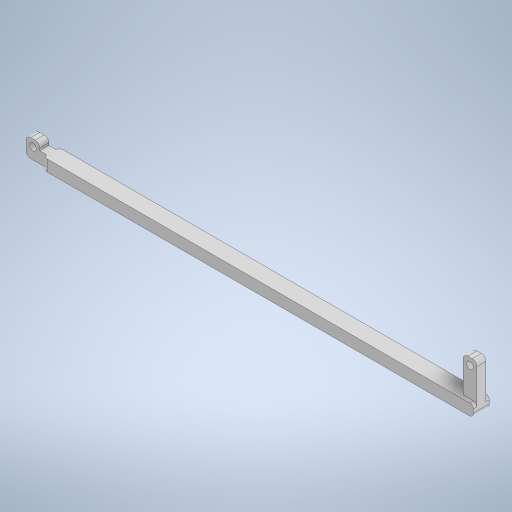
# Autodesk Inventor part: Brace_unequal
Saved by Autodesk Inventor 2024.3 (Build 283343000, 343)
## iProperties
Created: 2024-11-11
Part Number: Brace_unequal
Material: Generic
Document SubType Name: Modeling
Designer: magn1
Density: 1 g/cm^3
Appearance: Default
Author: magn1
Autodesk Inventor part; units mm, degrees
ref_plane "YZ Plane" through (0, 0, 0) normal (1, 0, 0) x (0, 1, 0)
ref_plane "XZ Plane" through (0, 0, 0) normal (0, 1, 0) x (-1, 0, 0)
ref_plane "XY Plane" through (0, 0, 0) normal (0, 0, 1) x (1, 0, 0)
sketch "Sketch1" plane through (0, 0, 0) normal (0, 1, 0) x (-1, 0, 0)
  line L0 (99.05, 3.5) -> (-99.05, 3.5)
  line L1 (-99.05, 3.5) -> (-99.05, -3.5)
  line L2 (-99.05, -3.5) -> (99.05, -3.5)
  line L3 (99.05, -3.5) -> (99.05, 3.5)
  line L4 (99.05, 3.5) -> (-99.05, -3.5) construction
  line L5 (-99.05, 3.5) -> (99.05, -3.5) construction
  point P0 (0, 0)
  dimension "d0" = 198.1
  dimension "d1" = 7
  constraints: 12 end point, 2 midpoint, 2 parallel, 1 horizontal, 1 perpendicular
  measures "d0" distance of L2.end L1.end
  measures "d1" distance of L1.end L0.end
extrude "Extrusion1" add sketch "Sketch1" along normal blind 5
sketch "Sketch2" plane through (0, 5, 0) normal (0, 1, 0) x (1, 0, 0)
  line L0 (99.05, -3.5) -> (99.05, 3.5) projected
  line L1 (99.05, 2) -> (93.05, 2)
  line L2 (93.05, 2) -> (93.05, -2)
  line L3 (93.05, -2) -> (99.05, -2)
  line L4 (99.05, -2) -> (99.05, 2)
  line L5 (99.05, 3.5) -> (-99.05, 3.5) projected
  point P0 (0, 0)
  dimension "d25" = 6
  dimension "d26" = 4
  dimension "d27" = 1.5
  constraints: 8 end point, 2 parallel, 1 horizontal, 1 perpendicular, 1 point on line
  measures "d25" distance of L3.end L2.end
  measures "d26" distance of L2.end L1.end
  measures "d27" distance between parallel lines of L5 L1
extrude "Extrusion2" add sketch "Sketch2" along normal blind 15.875
fillet "Fillet1" radius 2 2 edges at (99.05, 20.875, 0) (93.05, 20.875, 0)
sketch "Sketch4" plane through (0, 5, 0) normal (0, 1, 0) x (1, 0, 0)
  line L0 (99.05, 3.5) -> (-99.05, 3.5) projected
  line L1 (-99.05, 2) -> (-93.05, 2)
  line L2 (-93.05, 2) -> (-93.05, -2)
  line L3 (-93.05, -2) -> (-99.05, -2)
  line L4 (-99.05, -2) -> (-99.05, 2)
  line L5 (-99.05, 3.5) -> (-99.05, -3.5) projected
  point P0 (0, 0)
  dimension "d33" = 6
  dimension "d34" = 4
  dimension "d35" = 6
  dimension "d36" = 1.5
  constraints: 8 end point, 2 parallel, 1 horizontal, 1 perpendicular
  measures "d33" distance of L2.end L3.end
  measures "d34" distance of L1.end L2.end
  measures "d35" distance between parallel lines of L2 L5
  measures "d36" distance between parallel lines of L0 L1
extrude "Extrusion4" add sketch "Sketch4" along normal blind 3
fillet "Fillet2" radius 2 2 edges at (-93.05, 8, 0) (-99.05, 8, 0)
fillet "Fillet3" radius 2 2 edges at (99.05, 0, 0) (-99.05, 0, 0)
sketch "Sketch6" plane through (93.05, 5, 2) normal (0, 0, 1) x (1, 0, 0)
  line L0 (0, 15.875) -> (6, 15.875) construction
  line L1 (3, 15.875) -> (3, 12.875) construction
  line L2 (3, 15.875) -> (6, 15.875) construction
  circle A0 centre (3, 12.875) radius 1.5
  point P0 (-93.05, -5)
  dimension "d28" = 3
  dimension "d29" = 90
  dimension "d30" = 3
  constraints: 4 end point, 1 centre point, 1 coincident, 1 horizontal, 1 midpoint, 1 perpendicular, 1 vertical
  measures "d28" distance of L1.start L1.end
  measures "d29" angle of L1 L2
  measures "d30" diameter of A0
extrude "Extrusion6" cut sketch "Sketch6" against normal through all
sketch "Sketch7" plane through (-99.05, 5, 2) normal (0, 0, 1) x (1, 0, 0)
  line L0 (4, 3) -> (2, 3) construction
  line L1 (3, 3) -> (3, 0) construction
  line L2 (3, 3) -> (6, 3) construction
  circle A0 centre (3, 0) radius 1.5
  point P0 (99.05, -5)
  dimension "d57" = 1.5
  dimension "d37" = 3
  dimension "d38" = 90
  dimension "d39" = 3
  constraints: 4 end point, 1 centre point, 1 coincident, 1 horizontal, 1 midpoint, 1 perpendicular, 1 vertical
  measures "d37" distance of L1.start L1.end
  measures "d38" angle of L1 L2
  measures "d39" diameter of A0
sketch "Sketch8" plane through (0, 5, 0) normal (0, 1, 0) x (1, 0, 0)
  line L0 (-99.05, -3.5) -> (99.05, -3.5) projected
  line L1 (-93.05, -2) -> (-99.05, -2) projected
  line L2 (-99.05, -2) -> (-90.05, -2)
  line L3 (-90.05, -2) -> (-90.05, -3.5)
  line L4 (-90.05, -3.5) -> (-99.05, -3.5)
  line L5 (-99.05, -3.5) -> (-99.05, -2)
  line L6 (-99.05, 3.5) -> (-90.05, 3.5)
  line L7 (-90.05, 3.5) -> (-90.05, 2)
  line L8 (-90.05, 2) -> (-99.05, 2)
  line L9 (-99.05, 2) -> (-99.05, 3.5)
  point P0 (0, 0)
  dimension "d54" = 9
  dimension "d55" = 1.5
  dimension "d56" = 9
  dimension "d57" = 1.5
  constraints: 16 end point, 4 parallel, 2 horizontal, 2 perpendicular
  measures "d54" distance of L3.end L4.end
  measures "d55" distance of L2.end L3.end
  measures "d56" distance of L7.end L8.end
  measures "d57" distance of L6.end L7.end
extrude "Extrusion7" cut sketch "Sketch8" against normal through all
extrude "Extrusion8" cut sketch "Sketch7" against normal through all
fillet "Fillet5" radius 1.5 2 edges at (99.05, 5, 2.75) (99.05, 5, -2.75)
fillet "Fillet6" radius 2 2 edges at (-90.05, 2.5, 3.5) (-90.05, 2.5, -3.5)
body "Solid1"
